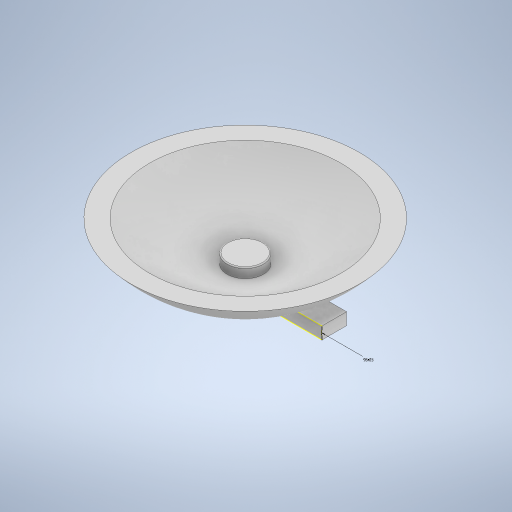
# Autodesk Inventor part: Dish final
Saved by Autodesk Inventor 2024 (Build 280153000, 153)
## iProperties
Created: 2023-07-01
Part Number: Dish final
Material: Generic
Document SubType Name: Modeling
Designer: hp
Density: 1 g/cm^3
Appearance: Default
Author: hp
Autodesk Inventor part; units mm, degrees
ref_plane "YZ Plane" through (0, 0, 0) normal (1, 0, 0) x (0, 1, 0)
ref_plane "XZ Plane" through (0, 0, 0) normal (0, 1, 0) x (-1, 0, 0)
ref_plane "XY Plane" through (0, 0, 0) normal (0, 0, 1) x (1, 0, 0)
sketch "Sketch1" plane through (0, 0, 0) normal (0, 0, 1) x (1, 0, 0)
  arc A0 (0, 0) -> (231.57, 111.025559) centre (0, 297.009717) ccw
  line L0 (0, 0) -> (0, 48.480564)
  arc A1 (0, 28.260564) -> (194, 111.025559) centre (0, 297.009717) ccw
  line L1 (231.57, 111.025559) -> (194, 111.025559)
  line L2 (36.83, 30.79616) -> (36.83, 48.480564)
  line L3 (36.83, 48.480564) -> (0, 48.480564)
  line L4 (36.83, 48.480564) -> (36.83, 48.480564)
  line L5 (34.83, 50.480564) -> (2, 50.480564)
  arc A2 (36.83, 48.480564) -> (34.83, 50.480564) centre (34.83, 48.480564) ccw
  line L6 (2, 50.480564) -> (0, 50.480564)
  line L7 (0, 50.480564) -> (0, 48.480564)
  point P0 (71.397957, -25.026885)
  point P1 (-122.602043, -107.79188)
  constraints: 16 end point, 7 point on circle, 3 centre point, 3 perpendicular, 3 vertical, 2 horizontal, 2 tangent, 1 point on line
revolve "Revolution1" add sketch "Sketch1" angle 360 about axis through (0, 0, 0) along (0, 1, 0)
sketch "Sketch2" plane through (0, 0, 0) normal (0, 0, 1) x (1, 0, 0)
  arc A0 (-231.57, 111.025559) -> (231.57, 111.025559) centre (0, 297.009717) ccw
  line L0 (0, 0) -> (180.848, 0)
  line L1 (180.848, 0) -> (180.848, 18.419799)
  line L2 (180.848, 18.419799) -> (180.848, 24.569296)
  line L3 (180.848, 24.569296) -> (118.283511, 24.569296)
  constraints: 8 end point, 2 vertical, 1 horizontal, 1 perpendicular, 1 point on circle, 1 tangent
extrude "Extrusion1" add sketch "Sketch2" along normal mid plane 50
sketch "Sketch3" plane through (0, 0, 25) normal (0, 0, 1) x (1, 0, 0)
  line L0 (180.848, 24.569296) -> (118.283511, 24.569296)
  line L1 (0, 0) -> (180.848, 0)
  arc A0 (180.848, 24.569296) -> (180.848, 0) centre (275.302486, 12.284648) ccw
  dimension "d8" = 95.25
  constraints: 2 point on circle, 1 centre point
  measures "d8" radius of A0
sketch "Sketch4" plane through (0, 0, 25) normal (0, 0, 1) x (1, 0, 0)
  line L0 (180.848, 24.569296) -> (180.848, 0) construction
  line L1 (180.848, 12.284648) -> (232.300575, 12.284648) construction
  point P0 (0, 0)
  constraints: 2 end point, 1 horizontal, 1 midpoint
body "Solid1"
